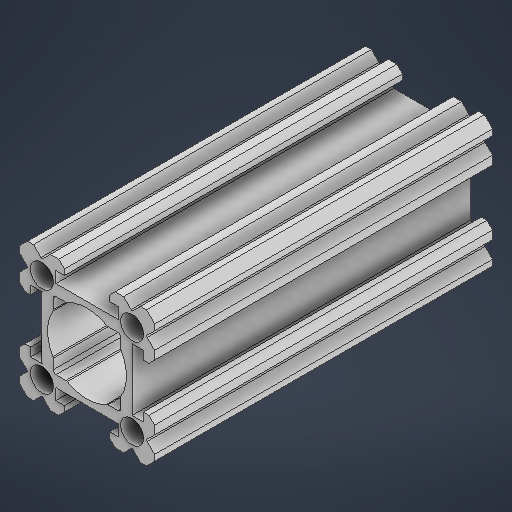
# Autodesk Inventor part: 1109-0024-0060
Saved by Autodesk Inventor 2026 (Build 300175050, 175E)
## iProperties
Created: 2025-11-11
Part Number: 1109-0024-0060
Material: Generic
Document SubType Name: Modeling
Designer: habbo
Density: 1 g/cm^3
Appearance: Default
Author: habbo
Autodesk Inventor part; units mm, degrees
ref_plane "YZ Plane" through (0, 0, 0) normal (1, 0, 0) x (0, 1, 0)
ref_plane "XZ Plane" through (0, 0, 0) normal (0, 1, 0) x (-1, 0, 0)
ref_plane "XY Plane" through (0, 0, 0) normal (0, 0, 1) x (1, 0, 0)
sketch "Sketch1" plane through (0, 0, 0) normal (0, 0, 1) x (1, 0, 0)
  line L0 (5.525, -10) -> (5.525, -8)
  line L1 (4, -10) -> (5.525, -10)
  line L2 (4, -11) -> (4, -10)
  line L3 (5, -12) -> (4, -11)
  line L4 (6.5, -12) -> (5, -12)
  line L5 (7.8232, -10.6768) -> (6.5, -12)
  arc A0 (8.1768, -10.6768) -> (7.8232, -10.6768) centre (8, -10.8536) ccw
  line L6 (9.5, -12) -> (8.1768, -10.6768)
  line L7 (10.5452, -12) -> (9.5, -12)
  arc A1 (10.5452, -12) -> (12, -10.5452) centre (0, 0) ccw
  line L8 (12, -10.5452) -> (12, -9.5)
  line L9 (10.6768, -8.1768) -> (12, -9.5)
  arc A2 (10.6768, -7.8232) -> (10.6768, -8.1768) centre (10.8535, -8) ccw
  line L10 (12, -6.5) -> (10.6768, -7.8232)
  line L11 (12, -6.5) -> (12, -5)
  line L12 (11, -4) -> (12, -5)
  line L13 (10, -4) -> (11, -4)
  line L14 (10, -5.525) -> (10, -4)
  line L15 (8, -5.525) -> (10, -5.525)
  line L16 (8, 5.525) -> (8, -5.525)
  line L17 (10, 5.525) -> (8, 5.525)
  line L18 (10, 4) -> (10, 5.525)
  line L19 (11, 4) -> (10, 4)
  line L20 (12, 5) -> (11, 4)
  line L21 (12, 5) -> (12, 6.5)
  line L22 (10.6768, 7.8232) -> (12, 6.5)
  arc A3 (10.6768, 8.1768) -> (10.6768, 7.8232) centre (10.8535, 8) ccw
  line L23 (12, 9.5) -> (10.6768, 8.1768)
  line L24 (12, 9.5) -> (12, 10.5452)
  arc A4 (12, 10.5452) -> (10.5452, 12) centre (0, 0) ccw
  line L25 (10.5452, 12) -> (9.5, 12)
  line L26 (8.1768, 10.6768) -> (9.5, 12)
  arc A5 (7.8232, 10.6768) -> (8.1768, 10.6768) centre (8, 10.8535) ccw
  line L27 (6.5, 12) -> (7.8232, 10.6768)
  line L28 (6.5, 12) -> (5, 12)
  line L29 (4, 11) -> (5, 12)
  line L30 (4, 10) -> (4, 11)
  line L31 (5.525, 10) -> (4, 10)
  line L32 (5.525, 8) -> (5.525, 10)
  line L33 (-5.525, 8) -> (5.525, 8)
  line L34 (-5.525, 10) -> (-5.525, 8)
  line L35 (-4, 10) -> (-5.525, 10)
  line L36 (-4, 11) -> (-4, 10)
  line L37 (-5, 12) -> (-4, 11)
  line L38 (-5, 12) -> (-6.5, 12)
  line L39 (-7.8232, 10.6768) -> (-6.5, 12)
  arc A6 (-8.1768, 10.6768) -> (-7.8232, 10.6768) centre (-8, 10.8535) ccw
  line L40 (-9.5, 12) -> (-8.1768, 10.6768)
  line L41 (-9.5, 12) -> (-10.5452, 12)
  arc A7 (-10.5452, 12) -> (-12, 10.5452) centre (0, 0) ccw
  line L42 (-12, 9.5) -> (-12, 10.5452)
  line L43 (-10.6768, 8.1768) -> (-12, 9.5)
  arc A8 (-10.6768, 7.8232) -> (-10.6768, 8.1768) centre (-10.8536, 8) ccw
  line L44 (-12, 6.5) -> (-10.6768, 7.8232)
  line L45 (-12, 5) -> (-12, 6.5)
  line L46 (-11, 4) -> (-12, 5)
  line L47 (-10, 4) -> (-11, 4)
  line L48 (-10, 5.525) -> (-10, 4)
  line L49 (-8, 5.525) -> (-10, 5.525)
  line L50 (-8, -5.525) -> (-8, 5.525)
  line L51 (-10, -5.525) -> (-8, -5.525)
  line L52 (-10, -4) -> (-10, -5.525)
  line L53 (-11, -4) -> (-10, -4)
  line L54 (-12, -5) -> (-11, -4)
  line L55 (-12, -6.5) -> (-12, -5)
  line L56 (-10.6768, -7.8232) -> (-12, -6.5)
  arc A9 (-10.6768, -8.1768) -> (-10.6768, -7.8232) centre (-10.8536, -8) ccw
  line L57 (-12, -9.5) -> (-10.6768, -8.1768)
  line L58 (-12, -10.5452) -> (-12, -9.5)
  arc A10 (-12, -10.5452) -> (-10.5452, -12) centre (0, 0) ccw
  line L59 (-9.5, -12) -> (-10.5452, -12)
  line L60 (-8.1768, -10.6768) -> (-9.5, -12)
  arc A11 (-7.8232, -10.6768) -> (-8.1768, -10.6768) centre (-8, -10.8536) ccw
  line L61 (-6.5, -12) -> (-7.8232, -10.6768)
  line L62 (-5, -12) -> (-6.5, -12)
  line L63 (-4, -11) -> (-5, -12)
  line L64 (-4, -10) -> (-4, -11)
  line L65 (-5.525, -10) -> (-4, -10)
  line L66 (-5.525, -8) -> (-5.525, -10)
  line L67 (5.525, -8) -> (-5.525, -8)
  arc A12 (6.0667, -3.4922) -> (6.0667, 3.4922) centre (0, 0) ccw
  arc A13 (6.0667, -3.4922) -> (6, -3.7417) centre (6.5, -3.7417) ccw
  line L68 (6, -5.5) -> (6, -3.7417)
  arc A14 (5.5, -6) -> (6, -5.5) centre (5.5, -5.5) ccw
  line L69 (5.5, -6) -> (3.7416, -6)
  arc A15 (3.7416, -6) -> (3.4922, -6.0667) centre (3.7416, -6.5) ccw
  arc A16 (-3.4922, -6.0667) -> (3.4922, -6.0667) centre (0, 0) ccw
  arc A17 (-3.4922, -6.0667) -> (-3.7417, -6) centre (-3.7417, -6.5) ccw
  line L70 (-3.7417, -6) -> (-5.5, -6)
  arc A18 (-6, -5.5) -> (-5.5, -6) centre (-5.5, -5.5) ccw
  line L71 (-6, -5.5) -> (-6, -3.7417)
  arc A19 (-6, -3.7417) -> (-6.0667, -3.4922) centre (-6.5, -3.7417) ccw
  arc A20 (-6.0667, 3.4922) -> (-6.0667, -3.4922) centre (0, 0) ccw
  arc A21 (-6.0667, 3.4922) -> (-6, 3.7417) centre (-6.5, 3.7417) ccw
  line L72 (-6, 3.7417) -> (-6, 5.5)
  arc A22 (-5.5, 6) -> (-6, 5.5) centre (-5.5, 5.5) ccw
  line L73 (-3.7417, 6) -> (-5.5, 6)
  arc A23 (-3.7417, 6) -> (-3.4922, 6.0667) centre (-3.7417, 6.5) ccw
  arc A24 (3.4922, 6.0667) -> (-3.4922, 6.0667) centre (0, 0) ccw
  arc A25 (3.4922, 6.0667) -> (3.7416, 6) centre (3.7416, 6.5) ccw
  line L74 (5.5, 6) -> (3.7416, 6)
  arc A26 (6, 5.5) -> (5.5, 6) centre (5.5, 5.5) ccw
  line L75 (6, 3.7417) -> (6, 5.5)
  arc A27 (6, 3.7417) -> (6.0667, 3.4922) centre (6.5, 3.7417) ccw
  circle A28 centre (-8, -8) radius 2.05
  circle A29 centre (8, -8) radius 2.05
  circle A30 centre (8, 8) radius 2.05
  circle A31 centre (-8, 8) radius 2.05
  point P0 (0, 0)
  point P1 (0, 0)
  constraints: 152 end point, 56 point on circle, 32 centre point
extrude "Extrusion1" add sketch "Sketch1" along normal mid plane 60
body "Solid1"
